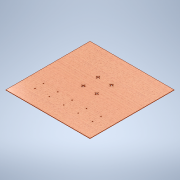
# Autodesk Inventor part: фанера
Saved by Autodesk Inventor 2020.1 (Build 241239000, 239)
## iProperties
Created: 2021-10-28
Part Number: фанера
Material: Древесина (дуб)
Document SubType Name: Modeling
Designer: Ni3na
Density: 0.76 g/cm^3
Appearance: Белый дуб — натуральный — с умеренным глянцем
Author: Ni3na
Autodesk Inventor part; units mm, degrees
ref_plane "YZ Plane" through (0, 0, 0) normal (1, 0, 0) x (0, 1, 0)
ref_plane "XZ Plane" through (0, 0, 0) normal (0, 1, 0) x (-1, 0, 0)
ref_plane "XY Plane" through (0, 0, 0) normal (0, 0, 1) x (1, 0, 0)
sketch "Эскиз1" plane through (0, 0, 0) normal (0, 1, 0) x (-1, 0, 0)
  line L0 (157.9407, 48.2001) -> (-242.0593, 48.2001)
  line L1 (-242.0593, 48.2001) -> (-242.0593, -351.7999)
  line L2 (-242.0593, -351.7999) -> (157.9407, -351.7999)
  line L3 (157.9407, -351.7999) -> (157.9407, 48.2001)
  point P0 (0, 0)
  dimension "d0" = 400
  dimension "d1" = 400
  constraints: 8 end point, 2 parallel, 1 horizontal, 1 perpendicular
  measures "d0" distance of L1.end L2.end
  measures "d1" distance of L0.end L1.end
extrude "Выдавливание1" add sketch "Эскиз1" along normal blind 2
sketch "Эскиз6" plane through (0, 0, 0) normal (0, -1, 0) x (1, 0, 0)
  line L0 (242.0593, -351.7999) -> (-157.9407, -351.7999) projected
  line L1 (-157.9407, -351.7999) -> (-157.9407, 48.2001) projected
  circle A0 centre (10.0593, -151.7939) radius 4
  circle A1 centre (42.0593, -186.9912) radius 47.5694
  circle A2 centre (74.0593, -151.7939) radius 4
  circle A3 centre (74.0593, -222.1885) radius 4
  circle A4 centre (10.0593, -222.1885) radius 4
  point P0 (0, 0)
  point P1 (42.0593, -351.7999)
  point P2 (-157.9407, -151.7999)
  point P3 (27.0149, -151.5386)
  dimension "d22" = 8
  dimension "d23" = 8
  dimension "d24" = 8
  dimension "d25" = 8
  dimension "d26" = 70.3946
  dimension "d27" = 64
  dimension "d28" = 70.3946
  dimension "d29" = 64
  constraints: 5 centre point, 4 point on circle, 2 coincident, 2 midpoint
  measures "d22" diameter of A0
  measures "d23" diameter of A2
  measures "d24" diameter of A3
  measures "d25" diameter of A4
  measures "d26" distance of A0.centre A4.centre
  measures "d27" distance of A0.centre A2.centre
  measures "d28" distance of A3.centre A2.centre
  measures "d29" distance of A4.centre A3.centre
extrude "Выдавливание3" cut sketch "Эскиз6" against normal blind 10 contours A0 A1 | A1 A0 | A2 A1 | A1 A2 | A4 A1 | A1 A4 | A3 A1 | A1 A3
sketch "Эскиз7" plane through (0, 0, 0) normal (0, -1, 0) x (1, 0, 0)
  circle A0 centre (178.7593, -26.7999) radius 2
  circle A1 centre (-94.4407, -26.7999) radius 2
  circle A2 centre (-26.1407, -26.7999) radius 2
  circle A3 centre (42.1593, -26.7999) radius 2
  circle A4 centre (110.4593, -26.7999) radius 2
  line L0 (242.0593, 48.2001) -> (242.0593, -351.7999) projected
  line L1 (-157.9407, 48.2001) -> (242.0593, 48.2001) projected
  circle A5 centre (178.7593, -66.7999) radius 2
  circle A6 centre (110.4593, -66.7999) radius 2
  circle A7 centre (42.0593, -66.7999) radius 2
  circle A8 centre (-26.1407, -66.7999) radius 2
  circle A9 centre (-94.4407, -66.7999) radius 2
  point P0 (0, 0)
  dimension "d33" = 4
  dimension "d34" = 4
  dimension "d35" = 4
  dimension "d36" = 4
  dimension "d37" = 4
  dimension "d38" = 63.3
  dimension "d39" = 75
  dimension "d40" = 68.3
  dimension "d41" = 68.3
  dimension "d42" = 68.3
  dimension "d43" = 68.3
  dimension "d44" = 4
  dimension "d45" = 4
  dimension "d46" = 4
  dimension "d47" = 4
  dimension "d48" = 40
  dimension "d49" = 40
  dimension "d50" = 40
  dimension "d51" = 40
  dimension "d52" = 40
  dimension "d77" = 4
  constraints: 10 centre point
  measures "d33" diameter of A0
  measures "d34" diameter of A1
  measures "d35" diameter of A2
  measures "d36" diameter of A3
  measures "d37" diameter of A4
  measures "d38" distance from line of A0.centre L0
  measures "d39" distance from line of L1 A0.centre
  measures "d40" distance of A4.centre A0.centre
  measures "d41" distance of A3.centre A4.centre
  measures "d42" distance of A2.centre A3.centre
  measures "d43" distance of A2.centre A1.centre
  measures "d44" diameter of A5
  measures "d45" diameter of A6
  measures "d46" diameter of A8
  measures "d47" diameter of A9
  measures "d48" distance of A0.centre A5.centre
  measures "d49" distance of A4.centre A6.centre
  measures "d50" vertical distance of A3.centre A7.centre
  measures "d51" distance of A2.centre A8.centre
  measures "d52" distance of A1.centre A9.centre
  measures "d77" diameter of A7
extrude "Выдавливание4" cut sketch "Эскиз7" against normal blind 10
sketch "Эскиз11" plane through (0, 0, 0) normal (0, -1, 0) x (1, 0, 0)
  circle A0 centre (74.0593, -222.1885) radius 4 projected
  circle A1 centre (74.0593, -222.1885) radius 7
  circle A2 centre (10.0593, -222.1885) radius 4 projected
  circle A3 centre (10.0593, -222.1885) radius 7
  circle A4 centre (10.0593, -151.7939) radius 4 projected
  circle A5 centre (10.0593, -151.7939) radius 7
  circle A6 centre (74.0593, -151.7939) radius 7
  circle A7 centre (81.0593, -222.1885) radius 1.5
  circle A8 centre (67.0593, -222.1885) radius 1.5
  circle A9 centre (74.0593, -229.1885) radius 1.5
  circle A10 centre (74.0593, -215.1885) radius 1.5
  circle A11 centre (74.0593, -158.7939) radius 1.5
  circle A12 centre (81.0593, -151.7939) radius 1.5
  circle A13 centre (74.0593, -144.7939) radius 1.5
  circle A14 centre (67.0593, -151.7939) radius 1.5
  circle A15 centre (17.0593, -151.7939) radius 1.5
  circle A16 centre (3.0593, -151.7939) radius 1.5
  circle A17 centre (10.0593, -158.7939) radius 1.5
  circle A18 centre (10.0593, -144.7939) radius 1.5
  circle A19 centre (10.0593, -215.1885) radius 1.5
  circle A20 centre (10.0593, -229.1885) radius 1.5
  circle A21 centre (3.0593, -222.1885) radius 1.5
  circle A22 centre (17.0593, -222.1885) radius 1.5
  point P0 (0, 0)
  dimension "d55" = 14
  dimension "d56" = 14
  dimension "d57" = 14
  dimension "d58" = 14
  dimension "d59" = 3
  dimension "d60" = 3
  dimension "d61" = 3
  dimension "d62" = 3
  dimension "d63" = 3
  dimension "d64" = 3
  dimension "d65" = 3
  dimension "d66" = 3
  dimension "d67" = 3
  dimension "d68" = 3
  dimension "d69" = 3
  dimension "d70" = 3
  dimension "d71" = 3
  dimension "d72" = 3
  dimension "d73" = 3
  dimension "d74" = 3
  constraints: 20 centre point, 16 point on circle, 3 coincident
  measures "d55" diameter of A1
  measures "d56" diameter of A3
  measures "d57" diameter of A5
  measures "d58" diameter of A6
  measures "d59" diameter of A7
  measures "d60" diameter of A8
  measures "d61" diameter of A9
  measures "d62" diameter of A10
  measures "d63" diameter of A11
  measures "d64" diameter of A12
  measures "d65" diameter of A13
  measures "d66" diameter of A14
  measures "d67" diameter of A15
  measures "d68" diameter of A16
  measures "d69" diameter of A17
  measures "d70" diameter of A18
  measures "d71" diameter of A19
  measures "d72" diameter of A20
  measures "d73" diameter of A22
  measures "d74" diameter of A21
extrude "Выдавливание5" cut sketch "Эскиз11" against normal blind 10 contours A1 A7 | A1 A7 | A10 A1 | A1 A10 | A9 A1 | A1 A9 | A8 A1 | A1 A8 | A3 A22 | A3 A22 | A19 A3 | A3 A19 | A20 A3 | A3 A20 | A21 A3 | A3 A21 | A5 A15 | A5 A15 | A18 A5 | A5 A18 | A17 A5 | A5 A17 | A16 A5 | A5 A16 | A6 A12 | A6 A12 | A13 A6 | A6 A13 | A11 A6 | A6 A11 | A14 A6 | A6 A14
